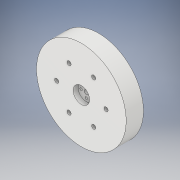
# Autodesk Inventor part: HA012
Saved by Autodesk Inventor 2017 SP1 (Build 210196100, 196)
## iProperties
Created: 2017-12-06
Part Number: HA012
Material: ABS Plastic
Document SubType Name: Modeling
Designer: Zach
Density: 1.06 g/cm^3
Appearance: CR White
Author: Zach
Autodesk Inventor part; units mm, degrees
ref_plane "YZ Plane" through (0, 0, 0) normal (1, 0, 0) x (0, 1, 0)
ref_plane "XZ Plane" through (0, 0, 0) normal (0, 1, 0) x (-1, 0, 0)
ref_plane "XY Plane" through (0, 0, 0) normal (0, 0, 1) x (1, 0, 0)
sketch "Sketch1" plane through (0, 0, 0) normal (0, 0, 1) x (1, 0, 0)
  circle A0 centre (0, 0) radius 54.5
  dimension "d0" = 109
  constraints: 1 centre point, 1 coincident
  measures "d0" diameter of A0
extrude "Extrusion1" add sketch "Sketch1" along normal blind 21
sketch "Sketch2" plane through (0, 0, 21) normal (0, 0, 1) x (1, 0, 0)
  circle A0 centre (0, 0) radius 10
  dimension "d3" = 20
  constraints: 1 centre point, 1 coincident
  measures "d3" diameter of A0
extrude "Extrusion2" cut sketch "Sketch2" against normal blind 6
sketch "Sketch3" plane through (0, 0, 15) normal (0, 0, 1) x (1, 0, 0)
  circle A0 centre (6.35, 0) radius 1.5
  circle A1 centre (0, 6.35) radius 1.5
  circle A2 centre (-6.35, 0) radius 1.5
  circle A3 centre (0, -6.35) radius 1.5
  point P0 (0, 0)
  dimension "d6" = 3
  dimension "d7" = 6.35
  dimension "d10" = 360
  constraints: 4 centre point, 1 horizontal alignment, 9 other
  measures "d6" diameter of A0
  measures "d7" distance of A0.centre point (0, 0)
extrude "Extrusion3" cut sketch "Sketch3" against normal through all
sketch "Sketch4" plane through (0, 0, 15) normal (0, 0, 1) x (1, 0, 0)
  circle A0 centre (0, 0) radius 2.5
  dimension "d14" = 5
  constraints: 1 centre point, 1 coincident
  measures "d14" diameter of A0
extrude "Extrusion4" cut sketch "Sketch4" against normal through all
sketch "Sketch5" plane through (0, 0, 0) normal (0, 0, -1) x (-1, 0, 0)
  circle A0 centre (6.35, 0) radius 1.5 projected
  circle A1 centre (6.35, 0) radius 3.5
  circle A2 centre (0, 6.35) radius 3.5
  circle A3 centre (-6.35, 0) radius 3.5
  circle A4 centre (0, -6.35) radius 3.5
  point P0 (0, 0)
  dimension "d17" = 7
  dimension "d20" = 360
  constraints: 4 centre point, 1 coincident, 9 other
  measures "d17" diameter of A1
extrude "Extrusion5" cut sketch "Sketch5" against normal blind 4 contours A0 | A1 | A2 | A3 | A4
sketch "Sketch6" plane through (0, 0, 0) normal (0, 0, -1) x (-1, 0, 0)
  circle A0 centre (-30, 0) radius 2.5
  circle A1 centre (-15, -25.9808) radius 2.5
  circle A2 centre (15, -25.9808) radius 2.5
  circle A3 centre (30, 0) radius 2.5
  circle A4 centre (15, 25.9808) radius 2.5
  circle A5 centre (-15, 25.9808) radius 2.5
  point P0 (0, 0)
  dimension "d24" = 5
  dimension "d25" = 30
  dimension "d28" = 360
  constraints: 6 centre point, 1 horizontal alignment, 13 other
  measures "d24" diameter of A0
  measures "d25" distance of A0.centre point (0, 0)
extrude "Extrusion6" cut sketch "Sketch6" against normal through all
body "Solid1"
